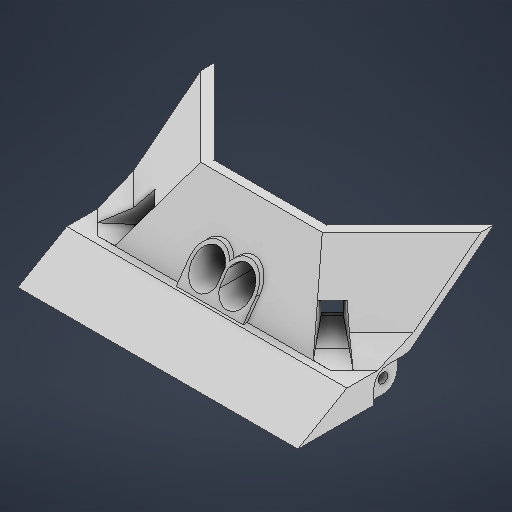
# Autodesk Inventor part: body-front
Saved by Autodesk Inventor 2025 (Build 290162000, 162)
## iProperties
Created: 2024-10-15
Part Number: body-front
Material: Všeobecné
Document SubType Name: Modeling
Designer: Simak
Density: 1 g/cm^3
Appearance: Výchozí
Author: Simak
Autodesk Inventor part; units mm, degrees
ref_plane "YZ Plane" through (0, 0, 0) normal (1, 0, 0) x (0, 1, 0)
ref_plane "XZ Plane" through (0, 0, 0) normal (0, 1, 0) x (-1, 0, 0)
sketch "Náčrt1" plane through (0, 0, 0) normal (1, 0, 0) x (0, 1, 0)
  line L0 (0, 48) -> (10, 30.6795)
  line L1 (10, 30.6795) -> (34, 13.8745)
  line L2 (10, 30.6795) -> (10, 28.1795)
  line L3 (10, 28.1795) -> (34, 11.3745)
  line L4 (34, 11.3745) -> (34, 13.8745)
  line L5 (34, 11.3745) -> (34, 1.3745)
  line L6 (34, 1.3745) -> (24, 1.3745)
  line L7 (24, 1.3745) -> (10, 11.1774)
  line L8 (10, 11.1774) -> (0, 11.1774)
  line L9 (0, 48) -> (0, 11.1774)
  point P0 (0, 0)
  point P1 (0, 0)
  dimension "d3" = 2.5
  dimension "d7" = 20
  dimension "d10" = 10
  dimension "d11" = 10
  dimension "d18" = 48
  dimension "d19" = 34
  dimension "d20" = 30
  dimension "d21" = 55
  dimension "d34" = 10
  constraints: 20 end point, 4 vertical, 2 parallel, 2 perpendicular, 2 point on line, 1 coincident, 1 vertical alignment
  measures "d3" distance of L0.end L2.end
  measures "d7" distance of L0.start L0.end
  measures "d10" distance of L3.end L5.end
  measures "d11" distance of L5.end L6.end
  measures "d18" distance of point (0, 0) L0.start
  measures "d19" distance from line of point (0, 0) L5
  measures "d20" angle of L9 L0
  measures "d21" angle of L9 L1
  measures "d34" distance of L7.end L8.end
extrude "Vysunutí1" add sketch "Náčrt1" along normal blind 49.5 contours L0 L2 L3 L5 L6 L7 L8 L9
sketch "Náčrt3" plane through (0, 0, 0) normal (-1, 0, 0) x (0, 0, 1)
  line L0 (48, 0) -> (11.1774, 0) projected
  line L1 (33.7254, 0) -> (33.7254, 4.2)
  line L2 (33.7254, 4.2) -> (22.3754, 4.2)
  line L3 (30.6795, 10) -> (48, 0) projected
  line L4 (11.1774, 10) -> (1.3745, 24) projected
  line L5 (11.1774, 0) -> (11.1774, 10) projected
  line L6 (48, 0) -> (11.1774, 0) projected
  line L7 (30.6795, 10) -> (48, 0) projected
  line L8 (28.1795, 10) -> (30.6795, 10) projected
  line L9 (11.3745, 34) -> (28.1795, 10) projected
  line L10 (1.3745, 34) -> (11.3745, 34) projected
  line L11 (1.3745, 24) -> (1.3745, 34) projected
  line L12 (1.3745, 34) -> (11.3745, 34) projected
  line L13 (8.3226, 34) -> (25.1276, 10)
  line L14 (25.1276, 10) -> (28.1795, 10)
  line L15 (25.1276, 10) -> (25.1276, 4.2)
  point P0 (0, 0)
  point P1 (11.1774, 0)
  dimension "d24" = 4.2
  dimension "d25" = 11.35
  dimension "d26" = 3.5
  dimension "d27" = 2.5
  constraints: 10 end point, 3 point on line, 2 parallel, 2 perpendicular, 1 vertical
  measures "d24" distance of L1.start L1.end
  measures "d25" distance of L1.end L2.end
  measures "d26" distance from line of L3 L1.end
  measures "d27" distance between parallel lines of L13 L9
extrude "Vysunutí2" cut sketch "Náčrt3" against normal blind 47 contours L0 L5 L4 L11 L10 L13 L15 L2 L1
sketch "Náčrt5" plane through (49.5, 0, 0) normal (1, 0, 0) x (0, 0, -1)
  circle A0 centre (-16.1774, 5) radius 5
  line L0 (-11.1774, 0) -> (-11.1774, 10) projected
  line L1 (-48, 0) -> (-11.1774, 0) projected
  line L2 (-16.1774, 10) -> (-11.1774, 10)
  line L3 (-21.1774, 5) -> (-21.1774, 0)
  point P0 (0, 0)
  point P1 (-16.1774, 0)
  point P2 (-11.1774, 5)
  dimension "d33" = 10
  constraints: 4 end point, 4 tangent, 2 point on circle, 1 centre point, 1 perpendicular, 1 point on line
  measures "d33" diameter of A0
extrude "Vysunutí3" add sketch "Náčrt5" against normal blind 4.25
extrude "Vysunutí4" cut sketch "Náčrt5" against normal blind 1.75
extrude "Vysunutí6" cut sketch "Náčrt5" against normal up to next contours L0 L1 A0
sketch "Náčrt7" plane through (45.25, 0, 0) normal (-1, 0, 0) x (0, 0, 1)
  line L0 (11.1774, 10) -> (16.1774, 10) projected
  arc A0 (21.1774, 5) -> (16.1774, 10) centre (16.1774, 5) ccw projected
  line L1 (21.1774, 5) -> (21.1774, 0) projected
  line L2 (33.7254, 0) -> (21.1774, 0) projected
  line L3 (33.7254, 4.2) -> (33.7254, 0) projected
  line L4 (25.1276, 4.2) -> (33.7254, 4.2) projected
  line L5 (25.1276, 10) -> (25.1276, 4.2) projected
  line L6 (8.3226, 34) -> (25.1276, 10) projected
  line L7 (1.3745, 34) -> (8.3226, 34) projected
  line L8 (1.3745, 24) -> (1.3745, 34) projected
  line L9 (11.1774, 10) -> (1.3745, 24) projected
  line L10 (10.0303, 11.6383) -> (19.3909, 18.1927)
  point P0 (0, 0)
  dimension "d39" = 2
  constraints: 2 end point, 2 point on line, 1 perpendicular
  measures "d39" distance of L0.start L10.start
extrude "Vysunutí5" add sketch "Náčrt7" against normal up to next contours L9 L10 L6 L5 L4 L3 L2 L1 A0 L0
sketch "Náčrt8" plane through (47.75, 0, 0) normal (1, 0, 0) x (0, 0, -1)
  arc A0 (-16.1774, 0) -> (-11.1774, 5) centre (-16.1774, 5) ccw projected
  point P0 (0, 0)
  constraints: 1 coincident
hole "Díra1" at (47.75, 5, 16.1774) direction (-1, 0, 0) diameter 3.4 depth 2.5 tip angle 118
sketch "Náčrt9" plane through (0, 4.2, 25.1276) normal (0, -1, 0) x (1, 0, 0)
  line L0 (0, 0) -> (0, 8.5978) projected
  line L1 (0, 8.5978) -> (45.25, 8.5978) projected
  point P0 (0, -25.1276)
  point P1 (20, 2.5978)
  dimension "d51" = 20
  dimension "d52" = 6
  measures "d51" distance from line of L0 point (20, 2.598)
  measures "d52" distance from line of L1 point (20, 2.598)
hole "Díra2" at (20, 4.2, 27.7254) direction (0, 1, 0) diameter 3 depth 4.5
sketch "Náčrt10" plane through (49.5, 24, 1.3745) normal (0, 0, -1) x (-1, 0, 0)
  circle A0 centre (44.175, -7.675) radius 5.325
  line L0 (49.5, 10) -> (49.5, -14) projected
  line L1 (49.5, -14) -> (0, -14) projected
  line L2 (49.5, -14) -> (0, -14) projected
  line L3 (36.25, 2.2) -> (36.25, -16.8)
  line L4 (36.25, 2.2) -> (49.5, 2.2)
  line L5 (40.5, 2.2) -> (40.5, 4.7)
  line L6 (40.5, 4.7) -> (49.5, 4.7)
  line L7 (36.25, -16.8) -> (49.5, -16.8)
  line L8 (49.5, -14) -> (49.5, -24) projected
  circle A1 centre (44.175, -7.675) radius 6.5
  line L9 (37.675, -7.675) -> (37.675, -14)
  line L10 (44.175, -1.175) -> (49.5, -1.175)
  line L11 (36.25, -4.477) -> (34.175, -5.675)
  circle A2 centre (34.175, -8.175) radius 2.5
  circle A3 centre (34.175, -8.175) radius 1.25
  line L12 (34.175, -10.675) -> (36.25, -11.873)
  line L13 (49, -5.4222) -> (49, -9.9278)
  line L14 (49, -5.4222) -> (49.5, -5.4222)
  line L15 (49, -9.9278) -> (49.5, -9.9278)
  point P0 (49.5, -7.675)
  point P1 (49.5, -3.9475)
  point P2 (36.25, -14)
  point P3 (36.25, -6.7806)
  point P4 (36.25, -9.5694)
  dimension "d60" = 10.65
  dimension "d61" = 1
  dimension "d62" = 13.25
  dimension "d63" = 19
  dimension "d64" = 9.875
  dimension "d65" = 2.5
  dimension "d66" = 9
  dimension "d67" = 13
  dimension "d68" = 5
  dimension "d69" = 2.5
  dimension "d70" = 10
  dimension "d71" = 0.5
  dimension "d72" = 60
  dimension "d84" = 0.5
  constraints: 24 end point, 10 point on line, 6 perpendicular, 6 point on circle, 4 centre point, 3 tangent, 3 vertical, 2 coincident, 2 vertical alignment, 1 equal length, 1 horizontal
  measures "d60" diameter of A0
  measures "d61" distance edge to line of A0 L1
  measures "d62" distance between parallel lines of L0 L3
  measures "d63" distance of L3.start L3.end
  measures "d64" vertical distance of L3.start A0.centre
  measures "d65" distance of L5.start L5.end
  measures "d66" distance of L5.end L6.end
  measures "d67" diameter of A1
  measures "d68" diameter of A2
  measures "d69" diameter of A3
  measures "d70" horizontal distance of A0.centre A2.centre
  measures "d71" vertical distance of A1.centre A2.centre
  measures "d72" angle of L3 L12
  measures "d84" distance between parallel lines of L0 L13
extrude "Vysunutí7" add sketch "Náčrt10" against normal blind 32.5 contours A0 L13 | L0 L15 A0 | A0 L14 L0 | A0 L15 L0 A1 L1 L14 | L0 L1 A1 | A1 L1 L9 picked at (49.0919, -8.1846)
sketch "Náčrt11" plane through (49.5, 0, 0) normal (1, 0, 0) x (0, 0, -1)
  line L0 (-11.3745, 34) -> (-28.1795, 10) projected
  line L1 (-28.1795, 10) -> (-30.6795, 10) projected
  line L2 (-29.6795, 10) -> (-12.8745, 34)
  line L3 (-12.8745, 34) -> (-11.3745, 34)
  line L4 (-33.8745, 22.825) -> (-33.8745, 16.325) projected
  line L5 (-33.8745, 10) -> (-33.8745, 16.325) projected
  line L6 (-30.6795, 10) -> (-33.8745, 10) projected
  line L7 (-19.1993, 22.825) -> (-33.8745, 22.825) projected
  point P0 (0, 0)
  point P1 (-33.8745, 20.0525)
  point P2 (-20.6993, 22.825)
  dimension "d75" = 1.5
  constraints: 4 end point, 1 horizontal, 1 parallel, 1 point on line
  measures "d75" distance of L0.end L2.start
extrude "Vysunutí8" cut sketch "Náčrt11" against normal through all contours L2 L1 L6 L5 L4 L7
extrude "Vysunutí9" cut sketch "Náčrt10" against normal through all contours L13 A0 picked at (45.6158, -8.8688)
extrude "Vysunutí11" add sketch "Náčrt10" against normal up to next contours A1 L10 L0 | L10 A1 L9 L1 L3 A2 L4 L0 | L3 A2 L11 | L12 A2 L3 | A2 L3 | L3 A2 | A3
extrude "Vysunutí10" cut sketch "Náčrt10" against normal blind 11.5 contours A0 L13 | L0 L15 A0 | A0 L14 L0 | L13 A0 | A0 L15 L0 A1 L1 L14 | A1 L10 L0 | L0 L1 A1 | L10 A1 L9 L1 L3 A2 L4 L0 | A1 L1 L9 | L3 A2 L11 | L12 A2 L3 | A2 L3 picked at (36.3277, -8.4953)
extrude "Vysunutí12" cut sketch "Náčrt10" against normal blind 13 contours A0 L13 | L0 L15 A0 | A0 L14 L0 picked at (49.0919, -8.1846)
sketch "Náčrt12" plane through (13.25, 10, 12.8745) normal (1, 0, 0) x (0, 0, -1)
  line L0 (-9.9249, 3.325) -> (-6.4238, 8.325)
  line L1 (0, 3.325) -> (-9.9249, 3.325)
  line L2 (0, 3.325) -> (0, 4.4306)
  line L3 (11.5, 4.4306) -> (0, 4.4306)
  line L4 (11.5, 7.2194) -> (11.5, 4.4306)
  line L5 (11.5, 7.2194) -> (0, 7.2194)
  line L6 (0, 7.2194) -> (0, 8.325)
  line L7 (0, 8.325) -> (-6.4238, 8.325)
  line L8 (0, 2.127) -> (0, 3.325)
  line L9 (0, 3.325) -> (-9.9249, 3.325)
  line L10 (-10.7637, 2.127) -> (-9.9249, 3.325)
  line L11 (0, 2.127) -> (-10.7637, 2.127)
  line L12 (0, 8.325) -> (0, 9.523)
  line L13 (0, 9.523) -> (-5.585, 9.523)
  line L14 (-6.4238, 8.325) -> (-5.585, 9.523)
  line L15 (0, 8.325) -> (-6.4238, 8.325)
  line L16 (-12.253, 0) -> (-10.7637, 2.127)
  line L17 (-10.7637, 2.127) -> (-9.9249, 3.325)
  line L18 (-9.9249, 3.325) -> (-6.4238, 8.325)
  line L19 (-6.4238, 8.325) -> (-5.585, 9.523)
  line L20 (-5.585, 9.523) -> (-0.9097, 16.2)
  line L21 (4.5519, 24) -> (-0.9097, 16.2)
  line L22 (4.5519, 24) -> (-6.5164, 8.1927)
  line L23 (-6.5164, 8.1927) -> (-12.253, 0)
  line L24 (0, 0) -> (0, 2.127)
  line L25 (0, 2.127) -> (-10.7637, 2.127)
  line L26 (-12.253, 0) -> (-10.7637, 2.127)
  line L27 (0, 0) -> (-12.253, 0)
  line L28 (0, 9.523) -> (0, 16.2)
  line L29 (0, 16.2) -> (-0.9097, 16.2)
  line L30 (-5.585, 9.523) -> (-0.9097, 16.2)
  line L31 (0, 9.523) -> (-5.585, 9.523)
  line L32 (11.5, 8.325) -> (-6.4238, 8.325)
  line L33 (11.5, 3.325) -> (-9.9249, 3.325)
  line L34 (11.5, 7.2194) -> (11.5, 4.4306)
  line L35 (11.5, 4.4306) -> (11.5, 7.2194)
  line L36 (11.5, 3.325) -> (11.5, 8.325)
  line L37 (-12.253, 0) -> (0.2387, 5.825)
  line L38 (0, 4.4306) -> (-9.1507, 4.4306)
  line L39 (11.5, 5.825) -> (-8.1743, 5.825)
  line L40 (-1.2638, 15.6942) -> (11.5, 8.325)
  point P0 (12.8745, -10)
  point P1 (11.5, 7.075)
  point P2 (11.5, 4.575)
  point P3 (-5.1226, 3.325)
  point P4 (-7.6917, 2.127)
  point P5 (-1.2638, 15.6942)
extrude "Vysunutí13" add sketch "Náčrt12" along normal blind 4.575 contours L0 L38 L37 L1 | L1 L37 L11 L10 | L0 L39 L37 L38 | L11 L37 L16 | L0 L7 L6 L5 L4 L39 | L14 L13 L12 L7 | L32 L36 L5 L6 | L12 L28 L40 L32 | L20 L40 L28 L13
ref_plane "Pracovní rovina1" through (17.825, 15.825, 1.3745) normal (0, 0.5, 0.8660254) x (-1, 0, 0)
sketch "Náčrt13" plane through (17.825, 15.825, 1.3745) normal (0, 0.5, 0.8660254) x (-1, 0, 0)
  ellipse E0 centre (2.5, 0) end of major axis (5, 0) minor radius 2.1651 (4.575, 1.2076) -> (0, 0) ccw projected
  ellipse E1 centre (2.5, 0) end of major axis (5, 0) minor radius 2.1651 (4.575, 1.2076) -> (0, 0) ccw projected
  line L0 (4.575, 1.2076) -> (4.575, -2.1651) projected
  line L1 (4.575, -2.1651) -> (0, -2.1651) projected
  line L2 (0, 0) -> (0, -2.1651) projected
  ellipse E2 centre (2.5, 0) end of major axis (5, 0) minor radius 2.1651 projected
  point P0 (17.825, 13.0176)
  point P1 (2.5, -2.1651)
  point P2 (4.575, -1.2076)
  constraints: 3 other
extrude "Vysunutí14" cut sketch "Náčrt13" along normal up to surface contours E2 L1 L2 | L0 L1 E2 surface through (0, 34, 8.3226) normal (0, 0.5735764, 0.819152)
fillet "Zaoblení1" radius 2.5 1 edges at (17.825, 12.9125, 18.8817)
sketch "Náčrt16" plane through (49.5, 24, 1.3745) normal (0, 0, -1) x (-1, 0, 0)
  circle A0 centre (34.175, -8.175) radius 1
  arc A1 (36.25, -6.7806) -> (31.675, -8.175) centre (34.175, -8.175) ccw projected
  point P0 (49.5, -24)
  dimension "d95" = 2
  constraints: 1 centre point, 1 concentric
  measures "d95" diameter of A0
extrude "Vysunutí15" cut sketch "Náčrt16" against normal blind 20
sketch "Náčrt17" plane through (0, 0, 0) normal (-1, 0, 0) x (0, 0, 1)
  line L0 (12.8745, 23.8589) -> (12.8745, 26.2) projected
  line L1 (12.8745, 26.2) -> (13.7842, 26.2) projected
  line L2 (14.6896, 24.9069) -> (13.7842, 26.2) projected
  line L3 (12.8745, 23.8589) -> (14.6896, 24.9069) projected
  line L4 (1.3745, 17.2194) -> (1.3745, 15.825) projected
  line L5 (12.8745, 23.8589) -> (1.3745, 17.2194) projected
  line L6 (12.8745, 23.8589) -> (14.6896, 24.9069) projected
  line L7 (15.3849, 23.9139) -> (14.6896, 24.9069) projected
  line L8 (15.3849, 23.9139) -> (1.3745, 15.825) projected
  line L9 (1.3745, 18.325) -> (1.3745, 15.825) projected
  line L10 (1.3745, 18.325) -> (14.1384, 25.6942)
  point P0 (0, 0)
  point P1 (12.8745, 24.9645)
  constraints: 2 end point, 1 parallel, 1 point on line
extrude "Vysunutí16" cut sketch "Náčrt17" against normal up to surface (13.25 mm away) contours L0 L1 L2 L10
extrude "Vysunutí17" add sketch "Náčrt17" against normal up to next contours L0 L10 L2 L3
sketch "Náčrt18" plane through (17.825, 10, 12.8745) normal (1, 0, 0) x (0, 0, -1)
  line L0 (-12.253, -5.8) -> (-20.8509, -5.8) projected
  line L1 (4.5519, 24) -> (-1.2638, 15.6942) projected
  line L2 (-0.9097, -5.8) -> (-0.9097, 16.2) construction
  point P0 (12.8745, -10)
  dimension "d102" = 22
  constraints: 2 end point, 1 coincident, 1 horizontal alignment, 1 point on line, 1 vertical
  measures "d102" distance of L2.start L2.end
sketch "Náčrt19" plane through (0, 4.2, 25.1276) normal (0, -1, 0) x (1, 0, 0)
  line L0 (17.825, -11.3434) -> (45.25, -11.3434) construction
  line L1 (45.25, -5.7366) -> (45.25, -15.0973) projected
  line L2 (20.4287, -12.0934) -> (26.7927, -18.4573)
  line L3 (26.0856, -19.1644) -> (19.7216, -12.8005)
  line L4 (19.7216, -12.8005) -> (20.4287, -12.0934)
  line L5 (26.0856, -19.1644) -> (26.7927, -18.4573)
  line L6 (17.825, -23.753) -> (17.825, -6.5762) projected
  line L7 (45.25, -5.7366) -> (45.25, 0) projected
  line L8 (26.7927, -18.4573) -> (45.25, 0) construction
  line L9 (19.4034, -12.6944) -> (26.0856, -19.3766)
  line L10 (26.0856, -19.3766) -> (27.0048, -18.4573)
  line L11 (27.0048, -18.4573) -> (20.3226, -11.7752)
  line L12 (19.4034, -12.6944) -> (20.3226, -11.7752)
  line L13 (20.6762, -13.9672) -> (19.6155, -15.0279)
  line L14 (19.6155, -15.0279) -> (17.825, -13.2373)
  line L15 (19.6155, -15.0279) -> (23.8582, -19.2705)
  line L16 (23.8582, -19.2705) -> (25.0249, -20.4372)
  line L17 (23.8582, -19.2705) -> (24.9188, -18.2098)
  line L18 (26.0856, -19.3766) -> (25.0249, -20.4372)
  line L19 (27.0048, -18.4573) -> (28.7726, -16.6896)
  line L20 (28.7726, -16.6896) -> (28.7726, 0)
  line L21 (0, 0) -> (45.25, 0) projected
  line L22 (17.825, -6.5762) -> (17.825, -2.8679) projected
  line L23 (17.825, -6.5762) -> (17.825, 0)
  point P0 (0, -25.1276)
  dimension "d103" = 45
  dimension "d104" = 1
  dimension "d105" = 9
  dimension "d106" = 0.75
  dimension "d110" = 0.15
  dimension "d111" = 0.3
  dimension "d112" = 1.5
  dimension "d113" = 1.5
  dimension "d114" = 1.5
  dimension "d115" = 2.5
  constraints: 38 end point, 10 point on line, 7 perpendicular, 3 parallel, 2 collinear, 1 horizontal, 1 vertical, 2 other
  measures "d103" angle of L0 L2
  measures "d104" distance between parallel lines of L3 L2
  measures "d105" distance of L2.start L2.end
  measures "d106" distance from line of L0 L2.start
  measures "d110" distance between parallel lines of L3 L9
  measures "d111" distance between parallel lines of L12 L4
  measures "d112" distance between parallel lines of L14 L9
  measures "d113" distance between parallel lines of L4 L13
  measures "d114" distance from line of L15.end L5
  measures "d115" distance of L10.end L19.end
extrude "Vysunutí19" add sketch "Náčrt19" against normal up to surface contours L6 L22 L23 L21 L20 L19 L11 L12 L9 L13 L14 surface through (0, 34, 8.3226) normal (0, 0.5735764, 0.819152)
sketch "Náčrt20" plane through (28.7726, 4.2, 25.1276) normal (1, 0, 0) x (0, 0, -1)
  line L0 (0, 5.8) -> (16.6896, 29.6352) projected
  line L1 (0, 0) -> (0, 5.8) projected
  line L2 (16.6896, 0) -> (0, 0) projected
  line L3 (16.6896, 0) -> (16.6896, 29.6352) projected
  line L4 (6.792, 15.5) -> (16.6896, 15.5)
  line L5 (18.4573, 32.1598) -> (16.805, 29.8) projected
  line L6 (16.6896, 29.6352) -> (16.805, 29.8) projected
  line L7 (16.6896, 0) -> (16.6896, 29.6352) projected
  line L8 (18.4573, 0) -> (16.6896, 0) projected
  line L9 (18.4573, 0) -> (18.4573, 32.1598) projected
  line L10 (16.6896, 15.5) -> (18.4573, 15.5)
  point P0 (25.1276, -4.2)
  point P1 (16.6896, 29.6352)
  dimension "d118" = 15.5
  constraints: 4 end point, 3 point on line, 2 perpendicular
  measures "d118" distance between parallel lines of L2 L4
extrude "Vysunutí20" cut sketch "Náčrt20" against normal up to surface (10.9476 mm away) contours L0 L3 L4 | L6 L5 L9 L10 L3
sketch "Náčrt21" plane through (28.7726, 4.2, 8.438) normal (0.7071068, 0, -0.7071068) x (-0.7071068, 0, -0.7071068)
  line L0 (2.5, 0) -> (2.5, 15.5) projected
  line L1 (2.5, 3.25) -> (1.75, 3.25)
  line L2 (1.75, 3.25) -> (1.75, 6.25)
  line L3 (2.5, 0) -> (0, 0) projected
  line L4 (2.5, 15.5) -> (0, 15.5) projected
  line L5 (1.75, 6.25) -> (0.5, 6.25)
  line L6 (0.5, 6.25) -> (0.5, 15.5)
  line L7 (1.75, 6.25) -> (2.5, 6.25)
  point P0 (26.3118, -4.2)
  dimension "d121" = 3.25
  dimension "d124" = 0.75
  dimension "d125" = 6.25
  dimension "d126" = 2
  constraints: 10 end point, 4 point on line, 2 horizontal, 2 perpendicular
  measures "d121" distance between parallel lines of L3 L1
  measures "d124" distance between parallel lines of L0 L2
  measures "d125" distance between parallel lines of L3 L5
  measures "d126" distance between parallel lines of L0 L6
extrude "Vysunutí21" cut sketch "Náčrt21" against normal up to surface (9.45 mm away) contours L1 L2 L7 L0
extrude "Vysunutí22" cut sketch "Náčrt21" against normal blind 7.5 contours L7 L5 L6 L4 L0
chamfer "Zkosení1" distance 0.75 angle 45 1 edges at (21.0114, 10.45, 12.6637)
sketch "Náčrt25" plane through (28.7726, 19.7, 18.3355) normal (0, 1, 0) x (1, 0, 0)
  line L0 (-0.3536, 10.2511) -> (-5.6569, 4.9478) projected
  line L1 (-5.6569, 4.9478) -> (-7.0711, 6.362) projected
  line L2 (-8.4499, 4.9832) -> (-7.0711, 6.362) projected
  line L3 (-9.3692, 5.9024) -> (-8.4499, 4.9832) projected
  line L4 (-8.0964, 7.1752) -> (-9.3692, 5.9024) projected
  line L5 (-9.157, 8.2358) -> (-8.0964, 7.1752) projected
  line L6 (-10.9476, 6.4453) -> (-9.157, 8.2358) projected
  line L7 (-10.9476, 6.4453) -> (-10.9476, 0) projected
  line L8 (0, 0) -> (-10.9476, 0) projected
  line L9 (0, 9.8975) -> (0, 0) projected
  line L10 (-0.3536, 10.2511) -> (0, 9.8975) projected
  line L11 (-5.6569, 4.9478) -> (20.7274, -21.4365) construction
  line L12 (20.7274, -12.3439) -> (20.7274, -29.6645) projected
  line L13 (-1.7324, 8.8722) -> (24.6519, -17.512) construction
  line L14 (-0.1768, 10.0743) -> (-1.5556, 8.6955) construction
  line L15 (-1.7324, 8.8722) -> (20.7274, -9.3154)
  line L16 (-5.6569, 4.9478) -> (20.7274, -27.6341)
  line L17 (20.7274, -9.8439) -> (20.7274, -12.3439) projected
  line L18 (20.7274, 6.961) -> (20.7274, -9.8439) projected
  line L19 (-16.9476, -9.8439) -> (20.7274, -9.8439) projected
  line L20 (-28.7726, -12.3439) -> (20.7274, -12.3439) projected
  line L21 (5.7722, -12.3439) -> (-8.3444, 5.0886)
  line L22 (20.7274, -6.7419) -> (-0.3104, 10.2942)
  line L23 (-0.3536, 10.2511) -> (-0.3104, 10.2942)
  line L24 (-1.7678, 11.6653) -> (0, 9.8975) projected
  line L25 (0, 9.8975) -> (0, 10.0429)
  point P0 (-28.7726, 18.3355)
  point P1 (0, 7.4694)
  point P2 (-1.6502, 0)
  point P3 (8.3457, -12.3439)
  point P4 (3.7477, -9.8439)
  point P5 (6.3213, -9.8439)
  dimension "d149" = 6
  dimension "d150" = 6
  dimension "d153" = 2
  dimension "d154" = 2
  constraints: 18 end point, 11 point on line, 5 parallel, 2 collinear, 1 midpoint, 1 perpendicular, 1 vertical
  measures "d149" angle of L13 L15
  measures "d150" angle of L16 L11
  measures "d153" distance between parallel lines of L21 L16
  measures "d154" distance between parallel lines of L22 L15
extrude "Vysunutí23" cut sketch "Náčrt25" against normal up to surface (9.7 mm away) contours L15 L9 L8 L16 L0 | L15 L18 L19 L16 L8 L9 | L19 L17 L20 L16
extrude "Vysunutí24" add sketch "Náčrt25" against normal up to surface (9.7 mm away) contours L23 L22 L25 L10 | L25 L22 L18 L15 L9 | L16 L8 L21 L2 L1 | L16 L19 L21 L8
ref_plane "Pracovní rovina7" through (6.4087, 10.45, -7.2438) normal (0.7071068, 0, -0.7071068) x (0, 1, 0)
sketch "Náčrt26" plane through (6.4087, 10.45, -7.2438) normal (0.7071068, 0, -0.7071068) x (0, 1, 0)
  line L0 (-0.45, 45.3315) -> (-0.45, 41.4259) projected
  line L1 (-0.45, 35.3419) -> (-0.45, 41.4259) projected
  line L2 (-0.45, 35.3419) -> (-0.45, 26.4024) projected
  line L3 (0, 26.4024) -> (-0.45, 26.4024) projected
  line L4 (0, 25.1524) -> (0, 26.4024) projected
  line L5 (-0.45, 49.7057) -> (-0.45, 28.6193) projected
  line L6 (-0.45, 55.1445) -> (-0.45, 57.286) projected
  line L7 (-0.45, 49.7057) -> (-0.45, 55.1445) projected
  line L8 (0, 26.4024) -> (-0.45, 49.7057)
  line L9 (-6.25, 38.7037) -> (-0.45, 38.7037) projected
  line L10 (-0.45, 38.7037) -> (-0.45, 39.6062) projected
  line L11 (-0.45, 39.6062) -> (-0.45, 41.4259) projected
  line L12 (-0.45, 41.4259) -> (-0.45, 50.355) projected
  line L13 (-0.45, 50.355) -> (-6.25, 50.355) projected
  line L14 (-6.25, 38.7037) -> (-6.25, 50.355) projected
  line L15 (-0.45, 37.5892) -> (1.801, 37.5892) projected
  line L16 (-0.45, 38.7037) -> (1.801, 37.5892) projected
  line L17 (-6.25, 38.7037) -> (-0.45, 38.7037) projected
  line L18 (-6.25, 26.9024) -> (-6.25, 38.7037) projected
  line L19 (-6.25, 26.9024) -> (-0.45, 26.9024) projected
  line L20 (-0.45, 26.9024) -> (-0.45, 28.6193) projected
  line L21 (-0.45, 28.6193) -> (-0.45, 35.3419) projected
  line L22 (-0.45, 35.3419) -> (-0.45, 37.5892) projected
  line L23 (-3, 25.1524) -> (0, 25.1524) projected
  line L24 (-3, 24.4024) -> (-3, 25.1524) projected
  line L25 (-6.25, 24.4024) -> (-3, 24.4024) projected
  line L26 (-6.25, 30.9626) -> (-6.25, 21.6024) projected
  line L27 (-0.45, 35.3419) -> (-0.45, 41.4259) projected
  line L28 (-0.45, 35.3419) -> (-0.45, 26.4024) projected
  line L29 (0, 26.4024) -> (-0.45, 26.4024) projected
  line L30 (0, 26.4024) -> (9.25, 26.4024) projected
  line L31 (9.25, 32.7341) -> (9.25, 26.4024) projected
  line L32 (9.25, 32.7341) -> (9.25, 36.6397) projected
  line L33 (9.25, 45.3315) -> (9.25, 36.6397) projected
  line L34 (9.25, 45.3315) -> (-0.45, 45.3315) projected
  line L35 (-0.45, 45.3315) -> (-0.45, 41.4259) projected
  line L36 (9.25, 32.7341) -> (9.25, 26.4024) projected
  line L37 (9.25, 26.4024) -> (14.318, 55.1445)
  line L38 (-0.45, 49.7057) -> (-0.45, 55.1445) projected
  line L39 (9.25, 55.1445) -> (-0.45, 55.1445) projected
  line L40 (9.25, 45.2463) -> (9.25, 55.1445) projected
  line L41 (9.25, 45.2463) -> (9.25, 40.4233) projected
  line L42 (9.25, 26.4024) -> (9.25, 40.4233) projected
  line L43 (0, 26.4024) -> (9.25, 26.4024) projected
  line L44 (0, 26.4024) -> (-0.45, 26.4024) projected
  line L45 (-0.45, 26.4024) -> (-0.45, 28.6193) projected
  line L46 (-0.45, 49.7057) -> (-0.45, 28.6193) projected
  line L47 (14.318, 55.1445) -> (9.25, 55.1445)
  line L48 (10.7731, 26.4024) -> (15.8411, 55.1445)
  line L49 (9.25, 26.4024) -> (9.25, 40.4233) projected
  line L50 (9.25, 26.4024) -> (10.7731, 26.4024)
  line L51 (14.318, 55.1445) -> (15.8411, 55.1445)
  point P0 (-10.45, 0.5905)
  point P1 (9.25, 45.2463)
  dimension "d157" = 10
  dimension "d160" = 1.5
  constraints: 12 end point, 3 horizontal, 1 horizontal alignment
  measures "d157" angle of L31 L37
  measures "d160" distance between parallel lines of L37 L48
extrude "Vysunutí25" add sketch "Náčrt26" against normal up to surface contours L40 L47 L37 L31 L32 L33 | L51 L48 L50 L37 surface through (32.5203, 19.7, 28.1795) normal (-0.777146, 0, 0.6293204)
extrude "Vysunutí26" cut sketch "Náčrt26" along normal up to surface contours L40 L47 L37 L31 L32 L33 surface through (37.1183, 19.7, 30.6795) normal (-0.777146, 0, 0.6293204)
extrude "Vysunutí27" add sketch "Náčrt26" along normal up to surface contours L40 L47 L37 L31 L32 L33 | L51 L48 L50 L37 surface through (28.4622, 19.7, 8.0413) normal (0.6293204, 0, -0.777146)
extrude "Vysunutí28" cut sketch "Náčrt26" against normal up to surface contours L40 L47 L37 L31 L32 L33 surface through (27.0402, 19.7, 9.4633) normal (0.6293204, 0, -0.777146)
extrude "Vysunutí29" add sketch "Náčrt26" along normal up to surface contours L34 L8 L16 L1 L0 | L5 L8 L34 | L8 L15 L1 L16 | L8 L3 L2 L1 L15 surface through (37.1183, 19.7, 30.6795) normal (-0.777146, 0, 0.6293204)
extrude "Vysunutí30" add sketch "Náčrt26" against normal up to surface contours L34 L8 L16 L1 L0 | L5 L8 L34 | L8 L15 L1 L16 | L8 L3 L2 L1 L15 surface through (27.0402, 19.7, 9.4633) normal (0.6293204, 0, -0.777146)
sketch "Náčrt27" plane through (49.5, 0, 0) normal (1, 0, 0) x (0, 0, -1)
  line L0 (-19.569, 22.2971) -> (-18.3162, 24.0863) projected
  line L1 (-18.3162, 24.0863) -> (-25.0774, 14.4302) projected
  line L2 (-11.3745, 34) -> (-25.0774, 14.4302) projected
  line L3 (-11.3745, 34) -> (-21.1406, 20.0525) projected
  line L4 (-21.1406, 20.0525) -> (-23.7507, 16.325) projected
  line L5 (-23.7507, 16.325) -> (-28.1795, 10) projected
  line L6 (-28.1795, 10) -> (-19.569, 22.2971) projected
  line L7 (-30.6795, 10) -> (-48, 0) projected
  line L8 (-30.6795, 10) -> (-48, 0) projected
  line L9 (-30.6795, 10) -> (-29.6795, 10) projected
  line L10 (-27.6509, 10) -> (-30.6795, 10) projected
  line L11 (-27.6509, 24.768) -> (-27.6509, 19.7) projected
  line L12 (-27.6509, 19.7) -> (-26.2289, 19.7) projected
  line L13 (-26.2289, 19.7) -> (-26.2289, 26.2911) projected
  line L14 (-26.2289, 26.2911) -> (-37.2696, 26.2911) projected
  line L15 (-37.2696, 26.2911) -> (-37.2696, 19.7) projected
  line L16 (-35.8476, 19.7) -> (-37.2696, 19.7) projected
  line L17 (-35.8476, 19.7) -> (-35.8476, 24.768) projected
  line L18 (-35.8476, 24.768) -> (-27.6509, 24.768) projected
  line L19 (-26.2289, 26.2911) -> (-18.3162, 24.0863) projected
  line L20 (-26.2289, 26.2911) -> (-37.2696, 26.2911) projected
  line L21 (-28.1795, 19.7) -> (-35.8476, 19.7) projected
  line L22 (-28.1795, 19.7) -> (-28.1795, 10.0845) projected
  line L23 (-25.2507, 16.325) -> (-29.6795, 10) projected
  line L24 (-37.2696, 6.1952) -> (-37.2696, 19.7)
  point P0 (0, 0)
  point P1 (-30.6795, 10)
  point P2 (-30.6795, 10)
  point P3 (-28.1795, 12.1422)
  constraints: 2 end point, 1 collinear, 1 point on line
extrude "Vysunutí31" cut sketch "Náčrt27" against normal up to surface (37.675 mm away)
extrude "Vysunutí32" cut sketch "Náčrt27" along normal through all contours L1 L5 L10 L23 L22 L21 L17 L18 L11 L12 L13 L19 L0 | L13 L12 L11 L18 L17 L16 L15 L14
ref_plane "Pracovní rovina8" through (45.25, 0, 25.1276) normal (-0.7071068, 0, 0.7071068) x (0, 1, 0)
sketch "Náčrt28" plane through (45.25, 0, 25.1276) normal (-0.7071068, 0, 0.7071068) x (0, 1, 0)
  line L0 (4.2, 11.6513) -> (10, 11.6513) projected
  line L1 (10, 11.6513) -> (10, 10.7488) projected
  line L2 (10, 10.7488) -> (10, 0.6493) projected
  line L3 (10, 0.6493) -> (10, 0) projected
  line L4 (10, 0) -> (4.2, 0) projected
  line L5 (4.2, 11.6513) -> (4.2, 0) projected
  line L6 (4.2, 0) -> (10, 10.0459)
  point P0 (0, 49.7644)
  dimension "d175" = 60
  constraints: 2 end point, 1 point on line
  measures "d175" angle of L4 L6
extrude "Vysunutí33" add sketch "Náčrt28" along normal up to next contours L6 L2 L3 L4
extrude "Vysunutí34" add sketch "Náčrt28" against normal up to surface contours L6 L2 L3 L4 surface through (28.4622, 19.7, 8.0413) normal (0.6293204, 0, -0.777146)
sketch "Náčrt29" plane through (6.4087, 10.45, -7.2438) normal (0.7071068, 0, -0.7071068) x (0, 1, 0)
  line L0 (12.0302, 42.1698) -> (10.8088, 35.2429) projected
  line L1 (5.875, 25.7463) -> (-0.45, 28.878) projected
  line L2 (-0.45, 28.878) -> (-0.45, 49.7057) projected
  line L3 (-0.364, 45.2545) -> (-0.45, 49.7057) projected
  line L4 (10.8088, 35.2429) -> (-0.364, 45.2545) projected
  line L5 (12.0302, 42.1698) -> (10.8088, 35.2429) projected
  line L6 (0.3049, 55.1445) -> (12.0302, 42.1698) projected
  line L7 (23.55, 43.6353) -> (0.3049, 55.1445) projected
  line L8 (23.55, 8.6335) -> (23.55, 43.6353) projected
  line L9 (23.55, 8.6335) -> (9.6025, 15.5392) projected
  ellipse E0 centre (5.875, 21.1501) end of major axis (-0.1681, 25.8349) minor radius 3.9071 (9.6025, 15.5392) -> (5.875, 25.7463) ccw projected
  line L10 (0.3049, 55.1445) -> (12.0302, 42.1698) projected
  line L11 (12.0302, 42.1698) -> (9.25, 26.4024) projected
  line L12 (0, 26.4024) -> (9.25, 26.4024) projected
  line L13 (0, 26.4024) -> (-0.45, 49.7057) projected
  line L14 (-0.45, 49.7057) -> (-0.45, 55.1445) projected
  line L15 (0.3049, 55.1445) -> (-0.45, 55.1445) projected
  line L16 (10.8088, 35.2429) -> (23.55, 23.826)
  line L17 (-0.45, 41.9747) -> (23.55, 20.4692)
  point P0 (-10.45, 0.5905)
  point P1 (-0.45, 49.7057)
  point P2 (-0.2981, 41.8386)
  point P3 (10.2977, 32.3441)
  dimension "d184" = 2.5
  constraints: 4 end point, 3 point on line, 1 collinear, 1 parallel, 1 other
  measures "d184" distance between parallel lines of L16 L17
extrude "Vysunutí35" cut sketch "Náčrt29" along normal blind 27 and the other way blind 32.5 contours L6 L7 L8 L16 L0 | L0 L4 L3 L14 L15 L6
extrude "Vysunutí36" add sketch "Náčrt29" along normal up to surface contours L11 L17 L13 L4 | L16 L8 L17 L11 surface through (49.5, 17, 24.6873) normal (1, 0, 0)
extrude "Vysunutí37" cut sketch "Náčrt29" against normal up to surface contours L11 L17 L13 L4 surface through (27.0402, 19.7, 9.4633) normal (0.6293204, 0, -0.777146)
sketch "Náčrt30" plane through (6.4087, 10.45, -7.2438) normal (-0.7071068, 0, 0.7071068) x (0.7071068, 0, 0.7071068)
  line L0 (22.0141, 23.55) -> (33.4379, 12.0137) projected
  line L1 (20.4692, 23.55) -> (22.0141, 23.55) projected
  line L2 (31.1655, 11.613) -> (20.4692, 23.55) projected
  line L3 (33.4379, 12.0137) -> (31.1655, 11.613) projected
  point P0 (0.5905, -10.45)
extrude "Vysunutí38" add sketch "Náčrt30" along normal up to surface surface through (0, 34, 8.3226) normal (0, 0.5735764, 0.819152)
ref_plane "Pracovní rovina10" through (13.0815, 0, -13.0815) normal (-0.7071068, 0, 0.7071068) x (0, 1, 0)
sketch "Náčrt32" plane through (13.0815, 0, -13.0815) normal (-0.7071068, 0, 0.7071068) x (0, 1, 0)
  line L0 (10.086, -44.664) -> (10, -49.1152) projected
  line L1 (10, -49.1152) -> (10, -56.6955) projected
  line L2 (21.2588, -34.6524) -> (10.086, -44.664) projected
  line L3 (34, -23.2355) -> (10.086, -44.664) projected
  line L4 (21.2588, -34.6524) -> (34, -23.2355) projected
  line L5 (10, -49.1152) -> (15.2323, -40.0525)
  point P0 (0, 0)
  point P1 (10.086, -44.664)
  point P2 (10.086, -44.664)
  dimension "d196" = 30
  constraints: 2 end point, 1 point on line
  measures "d196" angle of L1 L5
extrude "Vysunutí40" add sketch "Náčrt32" along normal up to surface surface through (27.0402, 19.7, 9.4633) normal (0.6293204, 0, -0.777146)
extrude "Vysunutí41" add sketch "Náčrt32" against normal up to surface surface through (49.5, 17, 24.6873) normal (1, 0, 0)
mirror "Zrcadlit1" about plane through (0, 17, 24.6873) normal (-1, 0, 0)
ref_plane "Pracovní rovina9" through (0, 0, 0) normal (-0.7071068, 0, 0.7071068) x (0, 1, 0)
